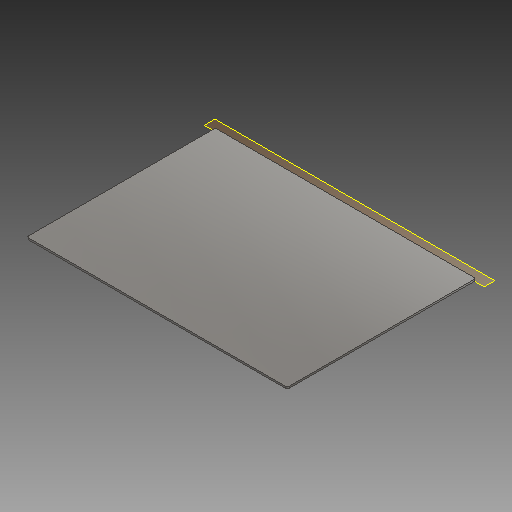
# Autodesk Inventor part: Deckel
Saved by Autodesk Inventor 2018 (Build 220112000, 112)
## iProperties
Created: 2017-10-08
Part Number: Deckel
Material: Edelstahl
Document SubType Name: Blech
Designer: jro
Density: 8 g/cm^3
Sheet Metal Rule: Standard_mm
Appearance: Halbpoliert
Author: jro
Autodesk Inventor part; units mm, degrees
ref_plane "YZ Plane" through (0, 0, 0) normal (1, 0, 0) x (0, 1, 0)
ref_plane "XZ Plane" through (0, 0, 0) normal (0, 1, 0) x (-1, 0, 0)
ref_plane "XY Plane" through (0, 0, 0) normal (0, 0, 1) x (1, 0, 0)
ref_plane "Arbeitsebene1" through (0, 0, 0) normal (0, 0, 1) x (1, 0, 0)
sketch "Skizze1" plane through (0, 0, 0) normal (0, 0, 1) x (1, 0, 0)
  line L0 (-141.4629, -2.7475) -> (141.4629, -2.7475)
  line L1 (141.4629, -6.7475) -> (-141.4629, -6.7475)
  arc A0 (-143.0858, -8.1175) -> (-141.4629, -6.7475) centre (-144.7619, -4.4856) ccw
  line L2 (-143.0858, -17.7475) -> (-143.0858, -8.1175)
  line L3 (143.0858, -17.7475) -> (-143.0858, -17.7475)
  line L4 (143.0858, -8.1175) -> (143.0858, -17.7475)
  arc A1 (141.4629, -6.7475) -> (143.0858, -8.1175) centre (144.7619, -4.4856) ccw
  line L5 (-141.4629, -218.7474) -> (141.4629, -218.7474)
  arc A2 (143.0858, -217.3774) -> (141.4629, -218.7474) centre (144.7619, -221.0093) ccw
  line L6 (143.0858, -207.7474) -> (143.0858, -217.3774)
  line L7 (-143.0858, -207.7474) -> (143.0858, -207.7474)
  line L8 (-143.0858, -217.3774) -> (-143.0858, -207.7474)
  arc A3 (-141.4629, -218.7474) -> (-143.0858, -217.3774) centre (-144.7619, -221.0093) ccw
  line L9 (146.5, -207.7104) -> (146.5, -217.7104)
  line L10 (146.5, -7.7845) -> (146.5, -17.7845)
  line L11 (-146.5, -216.7474) -> (-146.5, -8.7475)
  line L12 (146.5, -6.7475) -> (-146.5, -6.7475)
  line L13 (-146.5, -6.7475) -> (-146.5, -218.7474)
  line L14 (-146.5, -218.7474) -> (146.5, -218.7474)
  line L15 (146.5, -218.7474) -> (146.5, -6.7475)
  point P0 (0, 0)
  dimension "d0" = 0
  dimension "d1" = 0
  dimension "d2" = 0
  dimension "d3" = 0
  measures "d0" distance between parallel lines of L11 L13
  measures "d1" distance between parallel lines of L1 L12
  measures "d2" distance between parallel lines of L5 L14
  measures "d3" distance between parallel lines of L9 L15
extrude "Grobblech1" add sketch "Skizze1" along normal blind 2
fillet "Eckenrundung1" radius 2 4 edges at (146.5, -6.7475, 1) (-146.5, -6.7475, 1) (146.5, -218.7474, 1) (-146.5, -218.7474, 1)
equation "\"d4\" = Stärke"
equation "\"Biegeradius\" = Stärke"
equation "\"BreiteBiegungsfreistellung\" = Stärke"
equation "\"TiefeBiegungsfreistellung\" = 0.5 * Stärke"
equation "\"GrößeEckenfreistellung\" = 4 * Stärke"
equation "\"MinimalRest\" = 2 * Stärke"
equation "\"Übergangsradius\" = Biegeradius"
equation "\"JacobiRadiusGröße\" = Biegeradius"
equation "\"Abstandsgröße\" = Stärke"
equation "\"Stärke\" = 2"
